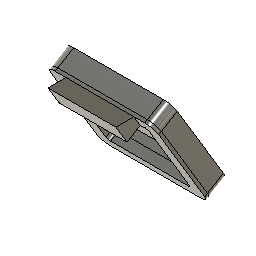
OLED Cover (Autodesk Fusion 360 design; units mm, degrees)
Autodesk Fusion 360 part; units mm, degrees
other "Base Mesh Feature1"
other "GenerateFaceGroups1"
other "GenerateFaceGroups2"
sketch "Sketch1" plane through (0, 0, 0) normal (0, 0, 1) x (1, 0, 0)
  line L0 (300, 270) -> (50, 270)
  line L1 (50, 270) -> (50, 120)
  line L2 (50, 120) -> (300, 120)
  line L3 (300, 120) -> (300, 270)
  line L4 (320, 350) -> (30, 350)
  line L5 (0, 320) -> (0, 30)
  line L6 (30, 0) -> (320, 0)
  line L7 (350, 30) -> (350, 320)
  arc A0 (350, 320) -> (320, 350) centre (320, 320) ccw
  arc A1 (30, 350) -> (0, 320) centre (30, 320) ccw
  arc A2 (0, 30) -> (30, 0) centre (30, 30) ccw
  arc A3 (320, 0) -> (350, 30) centre (320, 30) ccw
  dimension "d5" = 30
  constraint horizontal L0
  constraint vertical L1
  constraint horizontal L2
  constraint vertical L3
  constraint horizontal L4
  constraint vertical L5
  constraint horizontal L6
  constraint vertical L7
  constraint tangent L4 A0
  constraint tangent L7 A0
  constraint tangent L4 A1
  constraint tangent L5 A1
  constraint equal A0 A1
  constraint tangent L5 A2
  constraint tangent L6 A2
  constraint equal A0 A2
  constraint tangent L6 A3
  constraint tangent L7 A3
  constraint equal A0 A3
  measures "d5" radius of A0
  measures "d9" radius of L7.end
extrude "Extrude1" add sketch "Sketch1" along normal blind 10 makes body 1
sketch "Sketch2" plane through (0, 0, 10) normal (0, 0, 1) x (-1, 0, 0)
  line L0 (-300, -270) -> (-300, -120)
  line L1 (-300, -120) -> (-50, -120)
  line L2 (-50, -120) -> (-50, -270)
  line L3 (-50, -270) -> (-300, -270)
  arc A0 (-320, 0) -> (-350, -30) centre (-320, -30) ccw
  line L4 (-350, -30) -> (-350, -320)
  arc A1 (-350, -320) -> (-320, -350) centre (-320, -320) ccw
  line L5 (-320, -350) -> (-30, -350)
  arc A2 (-30, -350) -> (0, -320) centre (-30, -320) ccw
  line L6 (0, -320) -> (0, -30)
  arc A3 (0, -30) -> (-30, 0) centre (-30, -30) ccw
  line L7 (-30, 0) -> (-320, 0)
  line L8 (-300, -330) -> (-50, -330)
  arc A4 (-30, -330) -> (-20, -320) centre (-30, -320) ccw
  line L9 (-20, -300) -> (-20, -50)
  arc A5 (-20, -30) -> (-30, -20) centre (-30, -30) ccw
  line L10 (-50, -20) -> (-300, -20)
  arc A6 (-320, -20) -> (-330, -30) centre (-320, -30) ccw
  line L11 (-330, -50) -> (-330, -300)
  arc A7 (-330, -320) -> (-320, -330) centre (-320, -320) ccw
  arc A8 (-300, -20) -> (-330, -50) centre (-300, -50) ccw
  arc A9 (-20, -50) -> (-50, -20) centre (-50, -50) ccw
  arc A10 (-50, -330) -> (-20, -300) centre (-50, -300) ccw
  arc A11 (-330, -300) -> (-300, -330) centre (-300, -300) ccw
  dimension "d9" = 30
  constraint concentric A2 A4
  constraint concentric A3 A5
  constraint concentric A0 A6
  constraint concentric A1 A7
  constraint tangent L8 A7
  constraint tangent L10 A6
  constraint tangent A5 L10
  constraint tangent A4 L9
  constraint tangent L8 A4
  constraint tangent A6 L11
  constraint tangent L9 A5
  constraint tangent L11 A7
  constraint tangent L10 A8
  constraint tangent L11 A8
  constraint tangent L10 A9
  constraint tangent L9 A9
  constraint equal A8 A9
  constraint tangent L8 A10
  constraint tangent L9 A10
  constraint equal A8 A10
  constraint tangent L11 A11
  constraint tangent L8 A11
  constraint equal A8 A11
  measures "d9" radius of A8
extrude "Extrude2" add sketch "Sketch2" along normal blind 50 contours A0 L4 A1 L5 A2 L6 A3 L7 bodies 1
sketch "Sketch3" plane through (0, 0, 10) normal (0, 0, 1) x (-1, 0, 0)
  line L0 (-300, -330) -> (-50, -330)
  arc A0 (-50, -330) -> (-20, -300) centre (-50, -300) ccw
  line L1 (-20, -300) -> (-20, -50)
  arc A1 (-20, -50) -> (-50, -20) centre (-50, -50) ccw
  line L2 (-50, -20) -> (-300, -20)
  arc A2 (-300, -20) -> (-330, -50) centre (-300, -50) ccw
  line L3 (-330, -50) -> (-330, -300)
  arc A3 (-330, -300) -> (-300, -330) centre (-300, -300) ccw
  line L4 (-300, -270) -> (-300, -120)
  line L5 (-300, -120) -> (-50, -120)
  line L6 (-50, -120) -> (-50, -270)
  line L7 (-50, -270) -> (-300, -270)
  circle A4 centre (-70, -60) radius 12.4999
  line L8 (-30, 0) -> (-320, 0)
  line L9 (-320, -350) -> (-30, -350)
  line L10 (-175, 0) -> (-175, -350)
  line L11 (-350, -30) -> (-350, -320)
  line L12 (0, -320) -> (0, -30)
  line L13 (-350, -175) -> (0, -175)
  circle A5 centre (-280, -60) radius 12.4999
  circle A6 centre (-280, -290) radius 12.4999
  circle A7 centre (-70, -290) radius 12.4999
  constraint midpoint L8 L10.start
  constraint midpoint L9 L10.end
  constraint midpoint L11 L13.start
  constraint midpoint L12 L13.end
  constraint symmetric A4 L10 A5
  constraint symmetric A4 L13 A7
  constraint symmetric L13 A5 A6
extrude "Extrude3" add sketch "Sketch3" along normal blind 40 contours A4 | A5 | A6 | A7 bodies 1
other "MeshRemove1"
scale "Scale1" factor 0.1 about (300, 120, 0) bodies 1
sketch "Sketch4" plane through (0, 0, 6) normal (0, 0, 1) x (-1, 0, 0)
  arc A0 (-303, -138) -> (-300, -141) centre (-300, -138) ccw
  line L0 (-303, -138) -> (-303, -113)
  arc A1 (-300, -110) -> (-303, -113) centre (-300, -113) ccw
  line L1 (-300, -110) -> (-275, -110)
  arc A2 (-272, -113) -> (-275, -110) centre (-275, -113) ccw
  line L2 (-272, -113) -> (-272, -138)
  arc A3 (-275, -141) -> (-272, -138) centre (-275, -138) ccw
  line L3 (-275, -141) -> (-300, -141)
  line L4 (-273, -108) -> (-302, -108)
  arc A4 (-302, -108) -> (-305, -111) centre (-302, -111) ccw
  line L5 (-305, -111) -> (-305, -140)
  arc A5 (-305, -140) -> (-302, -143) centre (-302, -140) ccw
  line L6 (-302, -143) -> (-273, -143)
  arc A6 (-273, -143) -> (-270, -140) centre (-273, -140) ccw
  line L7 (-270, -140) -> (-270, -111)
  arc A7 (-270, -111) -> (-273, -108) centre (-273, -111) ccw
  arc A8 (-272.3, -113) -> (-275, -110.3) centre (-275, -113) ccw
  line L8 (-300, -110.3) -> (-275, -110.3)
  arc A9 (-300, -110.3) -> (-302.7, -113) centre (-300, -113) ccw
  line L9 (-302.7, -138) -> (-302.7, -113)
  arc A10 (-302.7, -138) -> (-300, -140.7) centre (-300, -138) ccw
  line L10 (-275, -140.7) -> (-300, -140.7)
  arc A11 (-275, -140.7) -> (-272.3, -138) centre (-275, -138) ccw
  line L11 (-272.3, -113) -> (-272.3, -138)
  arc A12 (-274, -113) -> (-275, -112) centre (-275, -113) ccw
  line L12 (-300, -112) -> (-275, -112)
  arc A13 (-300, -112) -> (-301, -113) centre (-300, -113) ccw
  line L13 (-301, -138) -> (-301, -113)
  arc A14 (-301, -138) -> (-300, -139) centre (-300, -138) ccw
  line L14 (-275, -139) -> (-300, -139)
  arc A15 (-275, -139) -> (-274, -138) centre (-275, -138) ccw
  line L15 (-274, -113) -> (-274, -138)
  dimension "d15" = 0.3
  dimension "d16" = 2
extrude "Extrude4" add sketch "Sketch4" against normal blind 2 separate body contours A8 L8 A9 L9 A10 L10 A11 L11 makes body 2
extrude "Extrude5" add sketch "Sketch4" along normal blind 1 separate body contours A0 L0 A1 L1 A2 L2 A3 L3 | L4 A4 L5 A5 L6 A6 L7 A7 | A8 L8 A9 L9 A10 L10 A11 L11 makes body 3
combine "Combine1" operation add target body 2 tool bodies 3
sketch "Sketch5" plane through (0, 0, 0) normal (1, 0, 0) x (0, 1, 0)
  line L0 (143, 7) -> (146, 12)
  line L1 (143, 7) -> (140, 7)
  line L2 (146, 12) -> (139, 12)
  line L3 (139, 12) -> (139, 7)
  line L4 (143, 7) -> (139, 7)
  point P0 (143, 7)
  point P1 (143, 7)
  constraint coincident P0 L0.start
  constraint parallel L1 L2
  constraint coincident L1 L3.end
  constraint perpendicular L1 L3
  constraint coincident P1 P0
move_body "Move1" bodies 2 1 to x (1, 0, 0) y (0, 1, 0) z (0, 0, 1) at (-287.5, 0, 0)
extrude "Extrude6" add sketch "Sketch5" along normal mid plane 22 bodies 2
move_body "Move2" bodies 1 2 to x (1, 0, 0) y (0, -0.515038, 0.857167) z (0, -0.857167, -0.515038) at (0, 163.6241, -92.5741)
move_face "OffsetFaces1" offset -0.6 4 faces at (9.2748, 101.6393, 3.4668) (-11.7484, 101.7347, 3.3079) (-9.3482, 91.3139, 23.2399) (11.6518, 91.3139, 23.2399) on bodies 1
